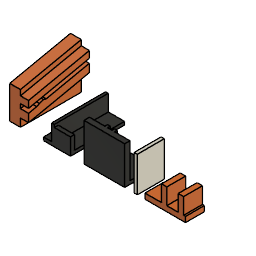
binstack-test-kit (Autodesk Fusion 360 design; units mm, degrees)
part number: 2026-08-18-20-08-31-071
part number: 2026-08-18-20-08-32-393
part number: 2026-08-18-20-08-32-488
part number: 2026-08-18-20-08-32-565
part number: 2026-08-18-20-08-32-684
part number: 2026-08-18-20-08-32-725
Autodesk Fusion 360 part; units mm, degrees
sketch "Sketch1" plane through (0, 0, 0) normal (1, 0, 0) x (0, 0, -1) in component "Купон полоза"
  line L0 (0, 0) -> (0, 45)
  line L1 (0, 45) -> (-33.765, 45)
  line L2 (-33.765, 45) -> (-24.2, 0)
  line L3 (-24.2, 0) -> (0, 0)
extrude "Extrude1" add sketch "Sketch1" along normal blind 8 makes body 1 in component "Купон полоза"
sketch "Sketch2" plane through (0, 0, 0) normal (1, 0, 0) x (0, 0, -1) in component "Купон полоза"
  line L0 (-6, 0) -> (-15.565, 45)
  line L1 (-15.565, 45) -> (-21.565, 45)
  line L2 (-21.565, 45) -> (-12, 0)
  line L3 (-12, 0) -> (-6, 0)
extrude "Extrude2" add sketch "Sketch2" along normal blind 6 from surface at 8 separate body makes body 2 in component "Купон полоза"
sketch "Sketch3" plane through (0, 0, 0) normal (1, 0, 0) x (0, 0, -1) in component "Купон полоза"
  line L0 (-15.2, 0) -> (-24.765, 45)
  line L1 (-24.765, 45) -> (-29.765, 45)
  line L2 (-29.765, 45) -> (-20.2, 0)
  line L3 (-20.2, 0) -> (-15.2, 0)
extrude "Extrude3" add sketch "Sketch3" along normal blind 6 from surface at 8 separate body makes body 3 in component "Купон полоза"
sketch "Sketch4" plane through (0, 0, 0) normal (1, 0, 0) x (0, 0, -1) in component "Купон полоза"
  line L0 (-13.2753, 6) -> (-14.2753, 8)
  line L1 (-14.2753, 8) -> (-15.3381, 11)
  line L2 (-15.3381, 11) -> (-14.7632, 13)
  line L3 (-14.7632, 13) -> (-13.2753, 6)
extrude "Extrude4" add sketch "Sketch4" along normal blind 6 from surface at 8 separate body makes body 4 in component "Купон полоза"
combine "Combine1" operation add target body 1 tool bodies 2 3 4 in component "Купон полоза"
sketch "Sketch1 (2)" plane through (0, 0, 0) normal (0, 0, 1) x (1, 0, 0) in component "Слайдер с фланцем"
  line L0 (0, 0) -> (20, 0)
  line L1 (20, 0) -> (20, 40)
  line L2 (20, 40) -> (0, 40)
  line L3 (0, 40) -> (0, 0)
extrude "Extrude1'" add sketch "Sketch1 (2)" along normal blind 2.4 separate body makes body 5 in component "Слайдер с фланцем"
sketch "Sketch2 (2)" plane through (0, 0, 0) normal (0, 0, 1) x (1, 0, 0) in component "Слайдер с фланцем"
  line L0 (6, 0) -> (8, 0)
  line L1 (8, 0) -> (8, 40)
  line L2 (8, 40) -> (6, 40)
  line L3 (6, 40) -> (6, 0)
extrude "Extrude2'" add sketch "Sketch2 (2)" along normal blind 12 from surface at 2.4 separate body makes body 6 in component "Слайдер с фланцем"
sketch "Sketch3 (2)" plane through (0, 0, 0) normal (0, 0, 1) x (1, 0, 0) in component "Слайдер с фланцем"
  line L0 (6, 0) -> (20, 0)
  line L1 (20, 0) -> (20, 3)
  line L2 (20, 3) -> (6, 3)
  line L3 (6, 3) -> (6, 0)
extrude "Extrude3'" add sketch "Sketch3 (2)" along normal blind 10 from surface at 2.4 separate body makes body 7 in component "Слайдер с фланцем"
combine "Combine1'" operation add target body 5 tool bodies 6 7 in component "Слайдер с фланцем"
sketch "Sketch1 (3)" plane through (0, 0, 0) normal (0, 0, 1) x (1, 0, 0) in component "Купон паза перегородки"
  line L0 (0, 0) -> (30, 0)
  line L1 (30, 0) -> (30, 22)
  line L2 (30, 22) -> (0, 22)
  line L3 (0, 22) -> (0, 0)
extrude "Extrude1''" add sketch "Sketch1 (3)" along normal blind 2.4 separate body makes body 8 in component "Купон паза перегородки"
sketch "Sketch2 (3)" plane through (0, 0, 0) normal (0, 0, 1) x (1, 0, 0) in component "Купон паза перегородки"
  line L0 (0, 0) -> (30, 0)
  line L1 (30, 0) -> (30, 4)
  line L2 (30, 4) -> (0, 4)
  line L3 (0, 4) -> (0, 0)
extrude "Extrude2''" add sketch "Sketch2 (3)" along normal blind 28 separate body makes body 9 in component "Купон паза перегородки"
sketch "Sketch3 (3)" plane through (0, 0, 0) normal (0, 0, 1) x (1, 0, 0) in component "Купон паза перегородки"
  line L0 (11.4, 4) -> (13.4, 4)
  line L1 (13.4, 4) -> (13.4, 6)
  line L2 (13.4, 6) -> (11.4, 6)
  line L3 (11.4, 6) -> (11.4, 4)
extrude "Extrude3''" add sketch "Sketch3 (3)" along normal blind 25.6 from surface at 2.4 separate body makes body 10 in component "Купон паза перегородки"
sketch "Sketch4 (2)" plane through (0, 0, 0) normal (0, 0, 1) x (1, 0, 0) in component "Купон паза перегородки"
  line L0 (16.6, 4) -> (18.6, 4)
  line L1 (18.6, 4) -> (18.6, 6)
  line L2 (18.6, 6) -> (16.6, 6)
  line L3 (16.6, 6) -> (16.6, 4)
extrude "Extrude4'" add sketch "Sketch4 (2)" along normal blind 25.6 from surface at 2.4 separate body makes body 11 in component "Купон паза перегородки"
combine "Combine1''" operation add target body 8 tool bodies 9 10 11 in component "Купон паза перегородки"
sketch "Sketch1 (4)" plane through (0, 0, 0) normal (0, 0, 1) x (1, 0, 0) in component "Перегородка"
  line L0 (0, 0) -> (2.4, 0)
  line L1 (2.4, 0) -> (2.4, 20)
  line L2 (2.4, 20) -> (0, 20)
  line L3 (0, 20) -> (0, 0)
extrude "Extrude1'''" add sketch "Sketch1 (4)" along normal blind 26 separate body makes body 12 in component "Перегородка"
sketch "Sketch1 (5)" plane through (0, 0, 0) normal (0, 0, 1) x (1, 0, 0) in component "Башмак подставки"
  line L0 (0, 0) -> (30, 0)
  line L1 (30, 0) -> (30, 14)
  line L2 (30, 14) -> (0, 14)
  line L3 (0, 14) -> (0, 0)
extrude "Extrude1''''" add sketch "Sketch1 (5)" along normal blind 4 separate body makes body 13 in component "Башмак подставки"
sketch "Sketch2 (4)" plane through (0, 0, 0) normal (0, 0, 1) x (1, 0, 0) in component "Башмак подставки"
  line L0 (12.2, 0) -> (16.2, 0)
  line L1 (16.2, 0) -> (16.2, 14)
  line L2 (16.2, 14) -> (12.2, 14)
  line L3 (12.2, 14) -> (12.2, 0)
extrude "Extrude2'''" add sketch "Sketch2 (4)" along normal blind 12 from surface at 4 separate body makes body 14 in component "Башмак подставки"
sketch "Sketch3 (4)" plane through (0, 0, 0) normal (0, 0, 1) x (1, 0, 0) in component "Башмак подставки"
  line L0 (24.6, 0) -> (28.6, 0)
  line L1 (28.6, 0) -> (28.6, 14)
  line L2 (28.6, 14) -> (24.6, 14)
  line L3 (24.6, 14) -> (24.6, 0)
extrude "Extrude3'''" add sketch "Sketch3 (4)" along normal blind 12 from surface at 4 separate body makes body 15 in component "Башмак подставки"
combine "Combine1'''" operation add target body 13 tool bodies 14 15 in component "Башмак подставки"
component "Купон полоза" placed x (1, 0, 0) y (0, 1, 0) z (0, 0, 1) at (0, 0, 0)
component "Слайдер с фланцем" placed x (1, 0, 0) y (0, 1, 0) z (0, 0, 1) at (25, 0, 0)
component "Купон паза перегородки" placed x (1, 0, 0) y (0, 1, 0) z (0, 0, 1) at (55, 0, 0)
component "Перегородка" placed x (1, 0, 0) y (0, 1, 0) z (0, 0, 1) at (92, 0, 0)
component "Башмак подставки" placed x (1, 0, 0) y (0, 1, 0) z (0, 0, 1) at (100, 0, 0)
named bodies: "Тело"
